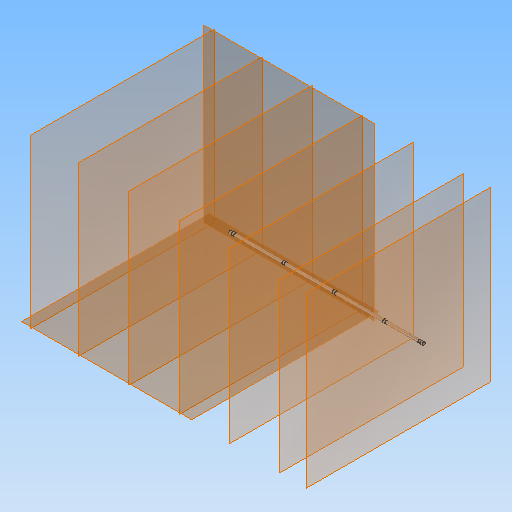
# Autodesk Inventor part: Pancake_Lever Shaft 2_4 Lanes
Saved by Autodesk Inventor 2018.1 (Build 221171000, 171)
## iProperties
Created: 2019-02-22
Part Number: Pancake_Lever Shaft 2_4 Lanes
Material: Stainless Steel
Document SubType Name: Modeling
Designer: James
Density: 8 g/cm^3
Appearance: Semi-Polished
Mass: 82.349 g
Surface Area: 69.7254 cm^2
Volume: 10.2936 cm^3
Author: James
Autodesk Inventor part; units mm, degrees
ref_plane "YZ Plane" through (0, 0, 0) normal (1, 0, 0) x (0, 1, 0)
ref_plane "XZ Plane" through (0, 0, 0) normal (0, 1, 0) x (-1, 0, 0)
ref_plane "XY Plane" through (0, 0, 0) normal (0, 0, 1) x (1, 0, 0)
derived "Pancake_Skeleton.ipt"
ref_plane "Ground" through (0, 0, 0) normal (0, 1, 0) x (-1, 0, 0)
ref_plane "Back" through (0, 0, 0) normal (0, 0, 1) x (1, 0, 0)
ref_plane "LHS" through (0, 0, 0) normal (1, 0, 0) x (0, 1, 0)
ref_plane "Lane 1" through (90, 0, 0) normal (1, 0, 0) x (0, 1, 0)
ref_plane "Lane 2" through (185, 0, 0) normal (1, 0, 0) x (0, 1, 0)
ref_plane "Lane 3" through (280, 0, 0) normal (1, 0, 0) x (0, 1, 0)
ref_plane "Lane 4" through (375, 0, 0) normal (1, 0, 0) x (0, 1, 0)
ref_plane "Lane 5" through (470, 0, 0) normal (1, 0, 0) x (0, 1, 0)
ref_plane "RHS" through (520, 0, 0) normal (1, 0, 0) x (0, 1, 0)
sketch "Sketch2" plane through (0, 0, 0) normal (0, 0, 1) x (1, 0, 0)
  line L0 (0, 3.6) -> (0, -0.6) projected
  line L1 (90, 3.6) -> (90, -0.6) projected
  line L2 (185, 3.6) -> (185, -0.6) projected
  line L3 (280, 3.6) -> (280, -0.6) projected
  line L4 (375, 3.6) -> (375, -0.6) projected
  line L5 (470, 3.6) -> (470, -0.6) projected
  line L6 (520, 3.6) -> (520, -0.6) projected
  line L7 (-81, 0) -> (486, 0) projected
  line L8 (40, 0) -> (405, 0)
  line L9 (405, 0) -> (405, 3)
  line L10 (405, 3) -> (40, 3)
  line L11 (40, 3) -> (40, 0)
  line L12 (-81, 0) -> (486, 0) projected
  point P0 (0, 0)
  dimension "d3" = 3
  dimension "d34" = 40
  dimension "d35" = 115
  constraints: 8 end point, 2 parallel, 1 horizontal, 1 perpendicular, 1 point on line
  measures "d3" distance of L8.end L9.end
  measures "d34" distance between parallel lines of L0 L11
  measures "d35" distance between parallel lines of L6 L9
revolve "Revolution1" add sketch "Sketch2" angle 360 about axis through (-10, 0, 0) along (1, 0, 0)
sketch "Sketch3" plane through (0, 0, 0) normal (0, 0, 1) x (1, 0, 0)
  line L0 (49, 3) -> (49.8, 3)
  line L1 (49.8, 3) -> (49.8, 2.85)
  line L2 (49.8, 2.85) -> (49, 2.85)
  line L3 (49, 2.85) -> (49, 3)
  line L4 (-9.96, 0) -> (59.76, 0) projected
  line L5 (40, -3) -> (40, 3) projected
  line L6 (90, 4.2) -> (90, -4.2) projected
  line L7 (-9.96, 0) -> (59.76, 0) projected
  line L8 (44.7, 3) -> (45.5, 3)
  line L9 (45.5, 3) -> (45.5, 2.85)
  line L10 (45.5, 2.85) -> (44.7, 2.85)
  line L11 (44.7, 2.85) -> (44.7, 3)
  line L12 (185, 4.2) -> (185, -4.2) projected
  line L13 (0, 4.2) -> (0, -4.2) projected
  point P0 (0, 0)
  dimension "d5" = 0.8
  dimension "d6" = 2.85
  dimension "d20" = 0.8
  dimension "d21" = 3.5
  dimension "d31" = 95
  dimension "d32" = 41
  dimension "d33" = 49
  constraints: 16 end point, 4 parallel, 3 horizontal alignment, 2 horizontal, 2 perpendicular
  measures "d5" distance of L0.start L0.end
  measures "d6" distance between parallel lines of L4 L2
  measures "d20" distance of L8.start L8.end
  measures "d21" distance of L0.start L8.end
  measures "d31" distance between parallel lines of L12 L6
  measures "d32" distance from line of L6 L0.start
  measures "d33" distance from line of L0.start L13
revolve "Revolution2" cut sketch "Sketch3" angle 360 about axis through (-10, 0, 0) along (1, 0, 0)
pattern_linear "Rectangular Pattern1" count 4 spacing 95 along (1, 0, 0) of "Revolution2"
sketch "Sketch4" plane through (0, 0, 0) normal (0, 0, 1) x (1, 0, 0)
  line L0 (15, 3) -> (15.8, 3)
  line L1 (15.8, 3) -> (15.8, 2.85)
  line L2 (15.8, 2.85) -> (15, 2.85)
  line L3 (15, 2.85) -> (15, 3)
  line L4 (40, -3) -> (40, 3) projected
  line L5 (-8, 0) -> (48, 0) projected
  line L6 (0, 4.2) -> (0, -4.2) projected
  line L7 (-8, 0) -> (48, 0) projected
  point P0 (0, 0)
  dimension "d14" = 2.85
  dimension "d15" = 0.8
  dimension "d17" = 15
  constraints: 8 end point, 2 parallel, 1 horizontal, 1 horizontal alignment, 1 perpendicular
  measures "d14" distance between parallel lines of L2 L5
  measures "d15" distance of L0.start L0.end
  measures "d17" distance from line of L0.start L6
revolve "Revolution3" [suppressed]
ref_plane "Mid Plane" through (260, 0, 0) normal (1, 0, 0) x (0, 1, 0)
mirror "Mirror1" [suppressed]
sketch "Sketch5" plane through (0, 0, 0) normal (0, 0, 1) x (1, 0, 0)
  line L0 (0, 4.2) -> (0, -4.2) projected
  line L1 (-9, 0) -> (54, 0) projected
  line L2 (40, 3) -> (45, 3)
  line L3 (45, 3) -> (45, 1.5)
  line L4 (45, 1.5) -> (40, 1.5)
  line L5 (40, 1.5) -> (40, 3)
  line L6 (44.7, 3) -> (44.7, -3) projected
  line L7 (40, -3) -> (40, 3) projected
  line L8 (40, -3) -> (40, 3) projected
  line L9 (-9, 0) -> (54, 0) projected
  point P0 (0, 0)
  dimension "d24" = 1.5
  dimension "d25" = 5
  constraints: 8 end point, 2 parallel, 1 coincident, 1 horizontal, 1 perpendicular, 1 point on line
  measures "d24" distance between parallel lines of L4 L1
  measures "d25" distance of L2.start L2.end
revolve "Revolution4" [suppressed]
mirror "Mirror2" [suppressed]
chamfer "Chamfer1" [suppressed]
fillet "Fillet1" [suppressed]
sketch "Sketch6" plane through (0, 0, 0) normal (0, 0, 1) x (1, 0, 0)
  line L0 (334.8, 3) -> (405, 3) projected
  line L1 (405, -3) -> (405, 3) projected
  line L2 (334.8, -3) -> (405, -3) projected
  line L3 (470, 4.2) -> (470, -4.2) projected
  line L4 (520, 4.2) -> (520, -4.2) projected
  line L5 (396.2, 3) -> (397, 3)
  line L6 (397, 3) -> (397, 2.85)
  line L7 (397, 2.85) -> (396.2, 2.85)
  line L8 (396.2, 2.85) -> (396.2, 3)
  line L9 (400, 3) -> (400.8, 3)
  line L10 (400.8, 3) -> (400.8, 2.85)
  line L11 (400.8, 2.85) -> (400, 2.85)
  line L12 (400, 2.85) -> (400, 3)
  line L13 (-100, 0) -> (600, 0) projected
  point P0 (0, 0)
  dimension "d36" = 2.85
  dimension "d37" = 3
  dimension "d38" = 0.8
  dimension "d39" = 0.8
  dimension "d41" = 120
  constraints: 16 end point, 4 parallel, 3 horizontal alignment, 2 horizontal, 2 perpendicular, 2 point on line
  measures "d36" distance between parallel lines of L11 L13
  measures "d37" distance of L9.start L5.end
  measures "d38" distance of L5.start L5.end
  measures "d39" distance of L9.start L9.end
  measures "d41" distance from line of L4 L11.end
revolve "Revolution5" cut sketch "Sketch6" angle 360 about axis through (-10, 0, 0) along (1, 0, 0)
chamfer "Chamfer2" distance 0.5 angle 45 2 edges at (405, -3, 0) (40, -3, 0)
equation "\"d20\" = d5"
equation "\"d39\" = d38"
body "Solid1"
